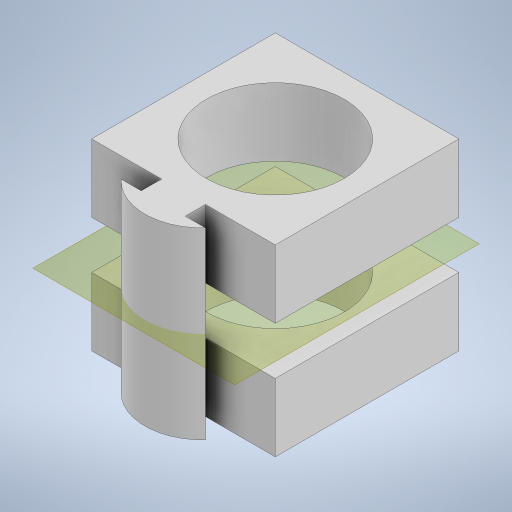
# Autodesk Inventor part: Connector MiniTec
Saved by Autodesk Inventor 2024 (Build 280153000, 153)
## iProperties
Created: 2024-01-18
Part Number: Connector MiniTec
Material: Generisch
Document SubType Name: Modeling
Designer: mariu
Density: 1 g/cm^3
Appearance: Vorgabe
Author: mariu
Autodesk Inventor part; units mm, degrees
ref_plane "YZ Plane" through (0, 0, 0) normal (1, 0, 0) x (0, 1, 0)
ref_plane "XZ Plane" through (0, 0, 0) normal (0, 1, 0) x (-1, 0, 0)
ref_plane "XY Plane" through (0, 0, 0) normal (0, 0, 1) x (1, 0, 0)
sketch "Skizze2" plane through (0, 0, 0) normal (0, 0, 1) x (1, 0, 0)
  line L0 (2.4, 0) -> (2.4, 7)
  line L1 (-2.4, 0) -> (-2.4, 7)
  line L2 (0, 0) -> (2.4, 0) construction
  line L3 (-2.4, 7) -> (2.4, 7)
  line L4 (-2.4, 0) -> (-4.6, 0)
  line L5 (2.4, 0) -> (4.6, 0)
  arc A0 (-4.6, 0) -> (4.6, 0) centre (0, 4.29) ccw
  point P0 (0, -2)
  dimension "d0" = 7
  dimension "d1" = 4.8
  dimension "d2" = 2.4
  dimension "d3" = 2.2
  dimension "d4" = 2
  constraints: 12 end point, 3 horizontal, 3 point on circle, 2 equal length, 2 vertical, 1 centre point, 1 parallel, 1 vertical alignment
  measures "d0" distance of L0.start L0.end
  measures "d1" distance between parallel lines of L1 L0
  measures "d2" distance of L2.start L0.start
  measures "d3" distance of L0.start L5.end
  measures "d4" distance of L2.start point (0, -2)
extrude "Extrusion1" add sketch "Skizze2" along normal blind 15
sketch "Skizze3" plane through (0, 0, 15) normal (0, 0, 1) x (1, 0, 0)
  line L0 (-2.4, 0) -> (-2.4, 2.2) construction
  line L1 (-2.4, 2.2) -> (-10, 2.2)
  line L2 (-2.4, 2.2) -> (10, 2.2)
  line L3 (-10, 2.2) -> (10, 2.2)
  line L4 (10, 2.2) -> (10, 7)
  line L5 (10, 7) -> (-10, 7)
  line L6 (-10, 7) -> (-10, 2.2)
  line L7 (-10, 7) -> (10, 7)
  line L8 (10, 7) -> (10, 22.2)
  line L9 (10, 22.2) -> (-10, 22.2)
  line L10 (-10, 22.2) -> (-10, 7)
  point P0 (0, 0)
  point P1 (2.4, 7)
  dimension "d7" = 2.2
  dimension "d8" = 20
  dimension "d9" = 10
  dimension "d10" = 20
  dimension "d39" = 20
  constraints: 22 end point, 4 horizontal, 4 parallel, 2 perpendicular, 1 horizontal alignment, 1 point on line, 1 vertical alignment
  measures "d7" distance of L0.start L0.end
  measures "d8" distance of L2.end L1.end
  measures "d9" horizontal distance of point (0, 0) L2.end
  measures "d10" distance between parallel lines of L6 L4
  measures "d39" distance between parallel lines of L2 L9
extrude "Extrusion2" add sketch "Skizze3" against normal blind 5
sketch "Skizze15" plane through (0, 0, 15) normal (0, 0, 1) x (1, 0, 0)
  circle A0 centre (0, 12.2) radius 7.5
  line L0 (-10, 22.2) -> (-10, 2.2) projected
  line L1 (10, 22.2) -> (-10, 22.2) projected
  point P0 (0, 0)
  dimension "d40" = 15
  dimension "d41" = 10
  dimension "d42" = 10
  constraints: 1 centre point
  measures "d40" diameter of A0
  measures "d41" distance from line of A0.centre L0
  measures "d42" distance from line of A0.centre L1
extrude "Extrusion12" cut sketch "Skizze15" against normal blind 5
sketch "Skizze16" plane through (0, 0, 0) normal (0, 0, -1) x (-1, 0, 0)
  line L0 (-10, 2.2) -> (-2.4, 2.2) projected
  line L1 (10, 22.2) -> (10, 2.2) projected
  line L2 (-10, 2.2) -> (10, 2.2)
  line L3 (10, 2.2) -> (10, 22.2)
  line L4 (10, 22.2) -> (-10, 22.2)
  line L5 (-10, 22.2) -> (-10, 2.2)
  point P0 (0, 0)
  point P1 (10, 2.2)
  constraints: 8 end point, 2 parallel, 1 horizontal, 1 perpendicular
extrude "Extrusion13" cut sketch "Skizze16" against normal blind 10
ref_plane "Arbeitsebene3" through (0, 0, 7.5) normal (0, 0, -1) x (-1, 0, 0)
mirror "Spiegeln2" about plane through (0, 0, 7.5) normal (0, 0, -1) of "Extrusion2", "Extrusion12"
sketch "Skizze18" plane through (0, 0, 7.5) normal (0, 0, -1) x (-1, 0, 0)
  line L0 (10, 2.2) -> (10, 22.2) projected
  line L1 (-10, 22.2) -> (-10, 2.2) projected
  line L2 (10, 2.2) -> (-10, 2.2)
  line L3 (-10, 2.2) -> (-10, 22.2)
  line L4 (-10, 22.2) -> (10, 22.2)
  line L5 (10, 22.2) -> (10, 2.2)
  point P0 (0, 0)
  point P1 (-10, 2.2)
  constraints: 8 end point, 2 parallel, 1 horizontal, 1 perpendicular
extrude "Extrusion14" cut sketch "Skizze18" along normal mid plane 5.2
sketch "Skizze19" plane through (0, 0, 15) normal (0, 0, 1) x (1, 0, 0)
  circle A0 centre (0, 12.2) radius 7.5 projected
  line L0 (-2.4, 2.2) -> (-2.4, 0) projected
  line L1 (-2.4, 0) -> (-4.6, 0) projected
  arc A1 (-4.6, 0) -> (4.6, 0) centre (0, 4.29) ccw projected
  line L2 (4.6, 0) -> (2.4, 0) projected
  line L3 (2.4, 0) -> (2.4, 2.2) projected
  line L4 (2.4, 2.2) -> (10, 2.2) projected
  line L5 (10, 2.2) -> (10, 22.2) projected
  line L6 (10, 22.2) -> (-10, 22.2) projected
  line L7 (-10, 22.2) -> (-10, 2.2) projected
  line L8 (-10, 2.2) -> (-2.4, 2.2) projected
  point P0 (0, 0)
extrude "Extrusion15" add sketch "Skizze19" along normal blind 2.5
mirror "Spiegeln3" about plane through (0, 0, 7.5) normal (0, 0, -1) of "Extrusion15"
ref_plane "Arbeitsebene4" through (0, 0, 7.5) normal (0, 0, -1) x (-1, 0, 0)
